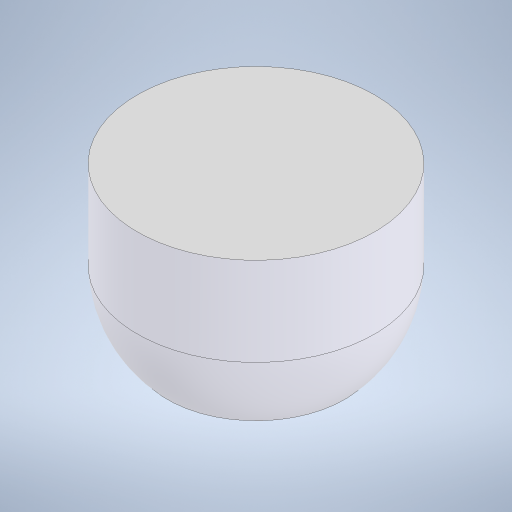
# Autodesk Inventor part: acoplamento_esfera
Saved by Autodesk Inventor 2023 (Build 270158000, 158)
## iProperties
Created: 2023-08-07
Part Number: acoplamento_esfera
Material: Genérico
Document SubType Name: Modeling
Designer: azeve
Density: 1 g/cm^3
Appearance: Padrão
Author: azeve
Autodesk Inventor part; units mm, degrees
ref_plane "YZ Plane" through (0, 0, 0) normal (1, 0, 0) x (0, 1, 0)
ref_plane "XZ Plane" through (0, 0, 0) normal (0, 1, 0) x (-1, 0, 0)
ref_plane "XY Plane" through (0, 0, 0) normal (0, 0, 1) x (1, 0, 0)
sketch "Esboço1" plane through (0, 0, 0) normal (1, 0, 0) x (0, 1, 0)
  arc A0 (-2.8528, -4.5384) -> (5.3606, 0) centre (0, 0) ccw
  line L0 (-2.8528, -4.5384) -> (-2.8528, -4.9924)
  line L1 (1.2086, -6.7016) -> (6.2047, -6.7016)
  line L2 (6.2047, -6.7016) -> (6.2047, 0)
  line L3 (0, 0) -> (-1.3092, 0)
  line L4 (-2.8528, 0) -> (7.2137, 0)
  arc A1 (-2.8528, -4.9924) -> (1.2086, -6.7016) centre (1.444, -0.4624) ccw
  constraints: 10 end point, 4 point on circle, 2 centre point, 2 horizontal, 2 vertical, 1 point on line
revolve "Revolução1" add sketch "Esboço1" angle 360 about axis through (0, -2.8528, 0) along (0, 1, 0)
